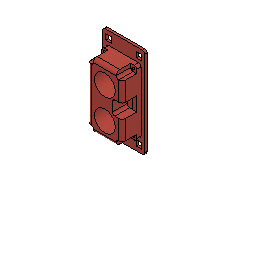
Ultrasonic Sensor Flat Mount (Autodesk Fusion 360 design; units mm, degrees)
Autodesk Fusion 360 part; units mm, degrees
sketch "Sketch1" plane through (0, 0, 1.778) normal (0, 0, 1) x (1, 0, 0)
  line L0 (10.414, -22.86) -> (10.414, 22.86)
  line L1 (10.414, 22.86) -> (-10.414, 22.86)
  line L2 (-10.414, 22.86) -> (-10.414, -22.86)
  line L3 (-10.414, -22.86) -> (10.414, -22.86)
  circle A0 centre (8.3312, -20.7772) radius 1.0668
  circle A1 centre (-8.3312, 20.7772) radius 1.0668
  line L4 (10.414, -22.86) -> (10.414, 22.86)
  line L5 (-10.414, -22.86) -> (10.414, -22.86)
  line L6 (-10.414, 22.86) -> (-10.414, -22.86)
  line L7 (10.414, 22.86) -> (-10.414, 22.86)
  circle A2 centre (0, 12.5374) radius 8.067
  circle A3 centre (0, -13.3706) radius 8.067
  line L8 (-10.914, 23.36) -> (-10.914, -23.36)
  line L9 (-10.914, -23.36) -> (10.914, -23.36)
  line L10 (10.914, -23.36) -> (10.914, 23.36)
  line L11 (10.914, 23.36) -> (-10.914, 23.36)
  circle A4 centre (0, -13.3706) radius 8.567
  circle A5 centre (0, 12.5374) radius 8.567
  line L12 (7.0383, 5.08) -> (7.0383, -5.08)
  line L13 (7.0383, -5.08) -> (10.0863, -5.08)
  line L14 (10.0863, -5.08) -> (10.0863, 5.08)
  line L15 (10.0863, 5.08) -> (7.0383, 5.08)
  line L16 (6.2883, 5.83) -> (6.2883, -5.83)
  line L17 (6.2883, -5.83) -> (10.8363, -5.83)
  line L18 (10.8363, -5.83) -> (10.8363, 5.83)
  line L19 (10.8363, 5.83) -> (6.2883, 5.83)
  line L20 (-14.414, 26.86) -> (-14.414, -26.86)
  line L21 (-14.414, -26.86) -> (14.414, -26.86)
  line L22 (14.414, -26.86) -> (14.414, 26.86)
  line L23 (14.414, 26.86) -> (-14.414, 26.86)
  line L24 (-5.914, 6) -> (-10.914, 6)
  line L25 (-10.914, 6) -> (-10.914, -6)
  line L26 (-10.914, -6) -> (-5.914, -6)
  line L27 (-5.914, -6) -> (-5.914, 6)
  line L28 (10.8363, 5.83) -> (14.414, 5.83)
  line L29 (14.414, 5.83) -> (14.414, -5.83)
  line L30 (14.414, -5.83) -> (10.8363, -5.83)
  line L31 (10.8363, -5.83) -> (10.8363, 5.83)
  dimension "d1" = 0.5
  dimension "d2" = 0.5
  dimension "d3" = 0.5
  dimension "d4" = 0.75
  dimension "d5" = 4
  dimension "d12" = 5
  dimension "d13" = 6
  dimension "d14" = 6
  measures "d1" distance of L2
  measures "d4" distance of L12
  measures "d5" distance of L2
  measures "d13" distance of origin
  measures "d14" distance of origin
extrude "Extrude1" add sketch "Sketch1" along normal blind 12.192 contours L0 L1 L2 L3 L4 L5 L6 L7 L16 L17 L19 L24 L26 L27 | L0 L2 L3 L4 L5 L6 L8 L9 L10 L17 L26 L30 | L0 L1 L2 L4 L6 L7 L8 L10 L11 L19 L24 L28 | L2 L6 L8 L24 L25 L26 | L2 L6 L24 L26 L27 | L8 L9 L10 L11 L20 L21 L22 L23 L25 L28 L30 | A0 | A1 makes body 1
fillet "Fillet1" radius 2 2 edges at (6.2883, 5.83, 7.874) (6.2883, -5.83, 7.874) on bodies 1
extrude "Extrude2" cut sketch "Sketch1" along normal blind 5 contours L2 L6 L8 L24 L25 L26 | L2 L6 L24 L26 L27 bodies 1
fillet "Fillet2" radius 2 2 edges at (-5.914, -6, 4.278) (-5.914, 6, 4.278) on bodies 1
extrude "Extrude3" add sketch "Sketch1" against normal blind 3.5 contours L8 L9 L10 L11 L20 L21 L22 L23 L25 L28 L30 | L10 L22 L28 L29 L30 bodies 1
sketch "Sketch2" plane through (0, 0, -1.722) normal (0, 0, -1) x (-1, 0, 0)
  line L0 (10.914, 23.36) -> (10.914, -23.36)
  line L1 (10.914, -23.36) -> (-10.914, -23.36)
  line L2 (-10.914, -23.36) -> (-10.914, 23.36)
  line L3 (-10.914, 23.36) -> (10.914, 23.36)
  line L4 (14.414, 26.86) -> (-14.414, 26.86)
  line L5 (-14.414, 26.86) -> (-14.414, -26.86)
  line L6 (-14.414, -26.86) -> (14.414, -26.86)
  line L7 (14.414, -26.86) -> (14.414, 26.86)
  circle A0 centre (-11.914, 24.36) radius 1
  circle A1 centre (11.914, 24.36) radius 1
  circle A2 centre (11.914, -24.36) radius 1
  circle A3 centre (-11.914, -24.36) radius 1
  line L8 (-14.414, -26.86) -> (-14.414, 26.86)
  line L9 (14.414, -26.86) -> (-14.414, -26.86)
  line L10 (14.414, 26.86) -> (14.414, -26.86)
  dimension "d18" = 2
  dimension "d19" = 2.5
  dimension "d20" = 2.5
  dimension "d21" = 2.5
  dimension "d22" = 2.5
  measures "d18" diameter of A3
  measures "d19" distance of L8
  measures "d20" distance of L9
  measures "d21" distance of L4
  measures "d22" distance of L10
extrude "Extrude4" cut sketch "Sketch2" against normal blind 15.692 contours A0 | A1 | A2 | A3 bodies 1
sketch "Sketch3" plane through (0, 0, 13.97) normal (0, 0, 1) x (1, 0, 0)
  circle A0 centre (-11.914, 24.36) radius 1
  circle A1 centre (-11.914, -24.36) radius 1
  circle A2 centre (11.914, 24.36) radius 1
  circle A3 centre (11.914, -24.36) radius 1
  circle A4 centre (0, -13.3706) radius 8.567
  circle A5 centre (0, 12.5374) radius 8.567
  line L0 (8.2883, 5.83) -> (14.414, 5.83)
  line L1 (14.414, 5.83) -> (14.414, 26.86)
  line L2 (14.414, 26.86) -> (-14.414, 26.86)
  line L3 (-14.414, 26.86) -> (-14.414, -26.86)
  line L4 (-14.414, -26.86) -> (14.414, -26.86)
  line L5 (14.414, -26.86) -> (14.414, -5.83)
  line L6 (14.414, -5.83) -> (8.2883, -5.83)
  arc A6 (6.2883, -3.83) -> (8.2883, -5.83) centre (8.2883, -3.83) ccw
  line L7 (6.2883, -3.83) -> (6.2883, 3.83)
  arc A7 (8.2883, 5.83) -> (6.2883, 3.83) centre (8.2883, 3.83) ccw
  circle A8 centre (-11.914, -24.36) radius 1
  circle A9 centre (11.914, -24.36) radius 1
  circle A10 centre (11.914, 24.36) radius 1
  circle A11 centre (-11.914, 24.36) radius 1
  line L8 (-14.414, 26.86) -> (-9.414, 26.86)
  line L9 (-9.414, 26.86) -> (-9.414, 21.86)
  line L10 (-9.414, 21.86) -> (-14.414, 21.86)
  line L11 (-14.414, 21.86) -> (-14.414, 26.86)
  line L12 (-14.414, 26.86) -> (-9.414, 21.86) construction
  line L13 (-9.414, 26.86) -> (-14.414, 21.86) construction
  line L14 (14.414, 26.86) -> (9.414, 26.86)
  line L15 (9.414, 26.86) -> (9.414, 21.86)
  line L16 (9.414, 21.86) -> (14.414, 21.86)
  line L17 (14.414, 21.86) -> (14.414, 26.86)
  line L18 (14.414, 26.86) -> (9.414, 21.86) construction
  line L19 (9.414, 26.86) -> (14.414, 21.86) construction
  line L20 (14.414, -26.86) -> (9.414, -26.86)
  line L21 (9.414, -26.86) -> (9.414, -21.86)
  line L22 (9.414, -21.86) -> (14.414, -21.86)
  line L23 (14.414, -21.86) -> (14.414, -26.86)
  line L24 (14.414, -26.86) -> (9.414, -21.86) construction
  line L25 (9.414, -26.86) -> (14.414, -21.86) construction
  line L26 (-14.414, -26.86) -> (-9.414, -26.86)
  line L27 (-9.414, -26.86) -> (-9.414, -21.86)
  line L28 (-9.414, -21.86) -> (-14.414, -21.86)
  line L29 (-14.414, -21.86) -> (-14.414, -26.86)
  line L30 (-14.414, -26.86) -> (-9.414, -21.86) construction
  line L31 (-9.414, -26.86) -> (-14.414, -21.86) construction
extrude "Extrude5" cut sketch "Sketch3" against normal blind 12 contours L1 L2 L14 L15 L16 L17 | L2 L3 L8 L9 L10 L11 | L4 L5 L20 L21 L22 L23 | L3 L4 L26 L27 L28 L29 bodies 1
fillet "Fillet3" radius 2 8 edges at (-9.414, 21.86, 7.97) (9.414, 21.86, 7.97) (9.414, -21.86, 7.97) (-9.414, -21.86, 7.97) (14.414, -26.86, 0.124) (14.414, 26.86, 0.124) (-14.414, 26.86, 0.124) (-14.414, -26.86, 0.124) on bodies 1
sketch "Sketch4" plane through (0, 0, -1.722) normal (0, 0, -1) x (-1, 0, 0)
  arc A0 (12.414, -26.86) -> (14.414, -24.86) centre (12.414, -24.86) ccw
  line L0 (14.414, -24.86) -> (14.414, 24.86)
  arc A1 (14.414, 24.86) -> (12.414, 26.86) centre (12.414, 24.86) ccw
  line L1 (12.414, 26.86) -> (-12.414, 26.86)
  arc A2 (-12.414, 26.86) -> (-14.414, 24.86) centre (-12.414, 24.86) ccw
  line L2 (-14.414, 24.86) -> (-14.414, -24.86)
  arc A3 (-14.414, -24.86) -> (-12.414, -26.86) centre (-12.414, -24.86) ccw
  line L3 (-12.414, -26.86) -> (12.414, -26.86)
  circle A4 centre (11.914, 24.36) radius 1
  circle A5 centre (11.914, -24.36) radius 1
  circle A6 centre (-11.914, 24.36) radius 1
  circle A7 centre (-11.914, -24.36) radius 1
  line L4 (10.914, 23.36) -> (10.914, -23.36)
  line L5 (10.914, -23.36) -> (-10.914, -23.36)
  line L6 (-10.914, -23.36) -> (-10.914, 23.36)
  line L7 (-10.914, 23.36) -> (10.914, 23.36)
  line L8 (-14.414, 0) -> (15, 0) construction
  line L9 (-12.7, -31.75) -> (12.7, -31.75)
  line L10 (12.7, -31.75) -> (12.7, 31.75)
  line L11 (12.7, 31.75) -> (-12.7, 31.75)
  line L12 (-12.7, 31.75) -> (-12.7, -31.75)
  line L13 (-12.7, -31.75) -> (12.7, 31.75) construction
  line L14 (12.7, -31.75) -> (-12.7, 31.75) construction
  line L15 (-14.986, -34.036) -> (-10.414, -34.036)
  line L16 (-10.414, -34.036) -> (-10.414, -29.464)
  line L17 (-10.414, -29.464) -> (-14.986, -29.464)
  line L18 (-14.986, -29.464) -> (-14.986, -34.036)
  line L19 (-14.986, -34.036) -> (-10.414, -29.464) construction
  line L20 (-10.414, -34.036) -> (-14.986, -29.464) construction
  line L21 (10.414, -34.036) -> (14.986, -34.036)
  line L22 (14.986, -34.036) -> (14.986, -29.464)
  line L23 (14.986, -29.464) -> (10.414, -29.464)
  line L24 (10.414, -29.464) -> (10.414, -34.036)
  line L25 (10.414, -34.036) -> (14.986, -29.464) construction
  line L26 (14.986, -34.036) -> (10.414, -29.464) construction
  line L27 (10.414, 34.036) -> (14.986, 34.036)
  line L28 (14.986, 34.036) -> (14.986, 29.464)
  line L29 (14.986, 29.464) -> (10.414, 29.464)
  line L30 (10.414, 29.464) -> (10.414, 34.036)
  line L31 (10.414, 34.036) -> (14.986, 29.464) construction
  line L32 (14.986, 34.036) -> (10.414, 29.464) construction
  line L33 (-14.986, 34.036) -> (-10.414, 34.036)
  line L34 (-10.414, 34.036) -> (-10.414, 29.464)
  line L35 (-10.414, 29.464) -> (-14.986, 29.464)
  line L36 (-14.986, 29.464) -> (-14.986, 34.036)
  line L37 (-14.986, 34.036) -> (-10.414, 29.464) construction
  line L38 (-10.414, 34.036) -> (-14.986, 29.464) construction
  line L39 (-17.5, -37.5) -> (17.5, -37.5)
  line L40 (17.5, -37.5) -> (17.5, 37.5)
  line L41 (17.5, 37.5) -> (-17.5, 37.5)
  line L42 (-17.5, 37.5) -> (-17.5, -37.5)
  line L43 (-17.5, -37.5) -> (17.5, 37.5) construction
  line L44 (17.5, -37.5) -> (-17.5, 37.5) construction
  line L45 (-14.414, -5.83) -> (-8.2883, -5.83)
  arc A8 (-8.2883, -5.83) -> (-6.2883, -3.83) centre (-8.2883, -3.83) ccw
  line L46 (-6.2883, -3.83) -> (-6.2883, 3.83)
  arc A9 (-6.2883, 3.83) -> (-8.2883, 5.83) centre (-8.2883, 3.83) ccw
  line L47 (-8.2883, 5.83) -> (-14.414, 5.83)
  line L48 (-10.914, -23.36) -> (-10.914, 23.36)
  dimension "d28" = 63.5
  dimension "d29" = 25.4
  dimension "d30" = 4.572
  dimension "d31" = 35
  dimension "d32" = 75
extrude "Extrude6" add sketch "Sketch4" along normal blind 2 separate body contours A0 A1 L1 A2 A3 L3 A4 A5 A6 A7 L4 L5 L6 L7 L10 L12 L45 L47 L48 | A0 A3 L3 L9 L10 L12 L16 L17 L23 L24 | A0 L0 A1 A4 A5 L10 | L2 A3 A7 L12 L45 | A1 L1 A2 L10 L11 L12 L29 L30 L34 L35 | L2 L12 L45 L47 | A2 L2 A6 L12 L47 | L6 L12 L45 L47 L48 | L4 L5 L6 L7 L45 A8 L46 A9 L47 L48 | L39 L40 L41 L42 makes body 2
fillet "Fillet4" radius 2 4 edges at (17.5, -37.5, -2.722) (-17.5, -37.5, -2.722) (-17.5, 37.5, -2.722) (17.5, 37.5, -2.722) on bodies 2
fillet "Fillet5" radius 3 5 edges at (14.414, -13.845, 13.97) (0, -26.86, 13.97) (-14.414, 0, 13.97) (14.414, 13.845, 13.97) (0, 26.86, 13.97) on bodies 1
sketch "Sketch5" plane through (0, 0, -1.722) normal (0, 0, 1) x (1, 0, 0)
  line L0 (14.986, 29.464) -> (10.414, 29.464)
  line L1 (10.414, 29.464) -> (10.414, 34.036)
  line L2 (10.414, 34.036) -> (14.986, 34.036)
  line L3 (14.986, 34.036) -> (14.986, 29.464)
  circle A0 centre (11.914, -24.36) radius 1
  line L4 (14.986, -29.464) -> (14.986, -34.036)
  line L5 (14.986, -34.036) -> (10.414, -34.036)
  line L6 (10.414, -34.036) -> (10.414, -29.464)
  line L7 (10.414, -29.464) -> (14.986, -29.464)
  line L8 (-10.414, -29.464) -> (-10.414, -34.036)
  line L9 (-10.414, -34.036) -> (-14.986, -34.036)
  line L10 (-14.986, -34.036) -> (-14.986, -29.464)
  line L11 (-14.986, -29.464) -> (-10.414, -29.464)
  circle A1 centre (11.914, 24.36) radius 1
  line L12 (10.914, -5.83) -> (8.2883, -5.83)
  arc A2 (6.2883, -3.83) -> (8.2883, -5.83) centre (8.2883, -3.83) ccw
  line L13 (6.2883, -3.83) -> (6.2883, 3.83)
  arc A3 (8.2883, 5.83) -> (6.2883, 3.83) centre (8.2883, 3.83) ccw
  line L14 (8.2883, 5.83) -> (10.914, 5.83)
  line L15 (10.914, 5.83) -> (10.914, -5.83)
  line L16 (-10.414, 29.464) -> (-14.986, 29.464)
  line L17 (-14.986, 29.464) -> (-14.986, 34.036)
  line L18 (-14.986, 34.036) -> (-10.414, 34.036)
  line L19 (-10.414, 34.036) -> (-10.414, 29.464)
  circle A4 centre (-11.914, 24.36) radius 1
  circle A5 centre (-11.914, -24.36) radius 1
  arc A6 (17.5, 35.5) -> (15.5, 37.5) centre (15.5, 35.5) ccw
  line L20 (15.5, 37.5) -> (-15.5, 37.5)
  arc A7 (-15.5, 37.5) -> (-17.5, 35.5) centre (-15.5, 35.5) ccw
  line L21 (-17.5, 35.5) -> (-17.5, -35.5)
  arc A8 (-17.5, -35.5) -> (-15.5, -37.5) centre (-15.5, -35.5) ccw
  line L22 (-15.5, -37.5) -> (15.5, -37.5)
  arc A9 (15.5, -37.5) -> (17.5, -35.5) centre (15.5, -35.5) ccw
  line L23 (17.5, -35.5) -> (17.5, 35.5)
  line L24 (-10.914, -23.36) -> (10.914, -23.36)
  line L25 (10.914, -23.36) -> (10.914, 23.36)
  line L26 (-10.914, 23.36) -> (-10.914, -23.36)
  line L27 (10.914, 23.36) -> (-10.914, 23.36)
extrude "Extrude7" cut sketch "Sketch5" against normal blind 1 contours L12 A2 L13 A3 L14 L24 L25 L26 L27 bodies 2
named bodies: "Ultrasoinc Top", "Ultrasonic Bottom"
